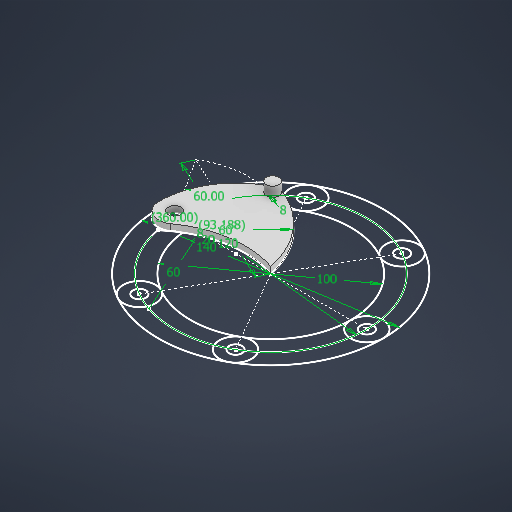
# Autodesk Inventor part: Shutter
Saved by Autodesk Inventor 2026.2 (Build 302298000, 298)
## iProperties
Created: 2025-12-30
Part Number: Shutter
Material: Generic
Document SubType Name: Modeling
Designer: Cobble
Density: 1 g/cm^3
Appearance: Default
Author: Cobble
Autodesk Inventor part; units mm, degrees
ref_plane "YZ Plane" through (0, 0, 0) normal (1, 0, 0) x (0, 1, 0)
ref_plane "XZ Plane" through (0, 0, 0) normal (0, 1, 0) x (-1, 0, 0)
ref_plane "XY Plane" through (0, 0, 0) normal (0, 0, 1) x (1, 0, 0)
sketch "Sketch1" plane through (0, 0, 0) normal (0, 0, 1) x (1, 0, 0)
  circle A0 centre (0, 0) radius 50
  circle A1 centre (0, 0) radius 60
  circle A2 centre (0, 0) radius 70
  circle A3 centre (-60, 0) radius 10
  circle A4 centre (-60, 0) radius 4
  line L0 (0, 0) -> (-60, 0) construction
  line L1 (0, 0) -> (-30, -51.9615) construction
  circle A5 centre (-30, -51.9615) radius 10
  circle A6 centre (-30, -51.9615) radius 4
  line L2 (0, 0) -> (30, -51.9615) construction
  circle A7 centre (30, -51.9615) radius 10
  circle A8 centre (30, -51.9615) radius 4
  line L3 (0, 0) -> (60, 0) construction
  circle A9 centre (60, 0) radius 10
  circle A10 centre (60, 0) radius 4
  line L4 (0, 0) -> (30, 51.9615) construction
  circle A11 centre (30, 51.9615) radius 10
  circle A12 centre (30, 51.9615) radius 4
  line L5 (0, 0) -> (-30, 51.9615) construction
  circle A13 centre (-30, 51.9615) radius 10
  circle A14 centre (-30, 51.9615) radius 4
  arc A15 (0, 0) -> (-39.6557, 45.027) centre (-58.8223, -11.8293) ccw
  arc A16 (0, 0) -> (-58.8223, -11.8293) centre (-19.1667, -56.8563) ccw
  arc A17 (-39.6557, 45.027) -> (-70, 0) centre (-21.4208, 0) ccw
  line L6 (0, 0) -> (60, 0) construction
  circle A18 centre (-39.521, 40.7393) radius 4
  arc A19 (-39.521, 40.7393) -> (-85.0417, 38.105) centre (-60, 0) ccw construction
  line L7 (-60, 0) -> (-85.0417, 38.105) construction
  line L8 (-60, 0) -> (-39.521, 40.7393) construction
  line L9 (-85.0417, 38.105) -> (0, 0) construction
  point P0 (-54.1667, -8.1223)
  point P1 (-38.1423, 44.4942)
  point P2 (-40.0141, 44.7088)
  point P3 (-41.1451, 44.3947)
  dimension "d42" = 140
  dimension "d43" = 20
  dimension "d40" = 100
  dimension "d41" = 120
  dimension "d44" = 8
  dimension "d47" = 360
  dimension "d49" = 60
  dimension "d50" = 60
  dimension "d58" = 8
  dimension "d59" = 60
  dimension "d60" = 93.1885
  constraints: 20 end point, 18 centre point, 11 point on circle, 9 coincident, 3 tangent, 2 horizontal, 1 horizontal alignment, 45 other
  measures "d40" diameter of A0
  measures "d41" diameter of A1
  measures "d44" diameter of A4
  measures "d49" radius of A15
  measures "d50" radius of A16
  measures "d58" diameter of A18
  measures "d59" angle of L8 L7
  measures "d60" distance of L7.end L5.start
extrude "Extrusion3" add sketch "Sketch1" along normal blind 4 contours A15 A16 A0 | A0 A3 A1 A18 A15 | A16 A3 A0 | A3 A1 A4 | A18 A1 | A3 A17 A18 A1 | A1 A4 A3 | A1 A18 picked at (-28.7442, 18.7739)
extrude "Extrusion4" add sketch "Sketch1" along normal blind 10 contours A18 A1 | A1 A18
body "Solid2"
